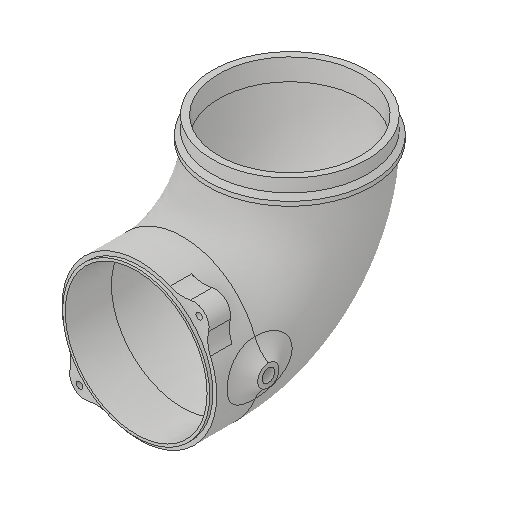
# Autodesk Inventor part: 3DP_PLA_Turbine_exhaust
Saved by Autodesk Inventor 2025 (Build 290162010, 162A)
## iProperties
Created: 2020-03-29
Part Number: 3DP_PLA_Turbine_exhaust
Material: Generic
Document SubType Name: Modeling
Designer: Andrzej
Density: 1 g/cm^3
Appearance: Default
Author: Andrzej
Autodesk Inventor part; units mm, degrees
ref_plane "XZ Plane" through (0, 0, 0) normal (0, 1, 0) x (-1, 0, 0)
ref_plane "XY Plane" through (0, 0, 0) normal (0, 0, 1) x (1, 0, 0)
sketch "Sketch1" plane through (0, 0, 0) normal (0, 0, 1) x (1, 0, 0)
  circle A0 centre (0, 0) radius 33
  circle A1 centre (0, 0) radius 36
  circle A2 centre (0, 0) radius 34.2
  dimension "d0" = 66
  dimension "d1" = 3
  dimension "d2" = 68.4
  constraints: 3 centre point, 2 coincident
  measures "d0" diameter of A0
  measures "d1" radial gap between concentric circles of A0 A1
  measures "d2" diameter of A2
extrude "Extrusion1" add sketch "Sketch1" along normal blind 1.5 contours A2
sketch "Sketch4" plane through (0, 0, 0) normal (1, 0, 0) x (0, 1, 0)
  line L0 (0, 0) -> (0, -20)
  line L1 (50, -70) -> (60, -70)
  arc A0 (0, -20) -> (50, -70) centre (50, -20) ccw
  dimension "d10" = 20
  dimension "d11" = 10
  dimension "d12" = 50
  dimension "d13" = 50
  dimension "d14" = 50
  constraints: 4 end point, 2 point on circle, 1 centre point, 1 horizontal, 1 vertical
  measures "d10" distance of L0.start L0.end
  measures "d11" distance of L1.start L1.end
  measures "d12" horizontal distance of L1.start L0.end
  measures "d13" horizontal distance of L1.start L0.end
  measures "d14" radius of A0
sweep "Sweep1" add profiles "Sketch1" path "Sketch4" path curves L0 A0 L1 contours A1 | A2
sketch "Sketch5" plane through (0, 0, 0) normal (0, 0, 1) x (1, 0, 0)
  circle A0 centre (0, 0) radius 36 projected
  circle A1 centre (0, 0) radius 34.2 projected
  line L0 (0, 0) -> (27.8105, 27.8105)
  line L1 (0, 0) -> (89.128, 0) construction
  line L2 (0, 0) -> (-27.8105, -27.8105)
  line L3 (0, 0) -> (71.454, 0) construction
  circle A2 centre (0, 0) radius 39.33
  circle A3 centre (27.8105, 27.8105) radius 1.5
  circle A4 centre (-27.8105, -27.8105) radius 1.5
  circle A5 centre (0, 0) radius 36 projected
  arc A6 (-29.9009, -20.0483) -> (-20.0483, -29.9009) centre (-25.4558, -25.4558) ccw
  arc A7 (29.9009, 20.0483) -> (20.0483, 29.9009) centre (25.4558, 25.4558) ccw
  dimension "d18" = 45
  dimension "d20" = 135
  dimension "d21" = 78.66
  dimension "d22" = 3
  dimension "d23" = 3
  dimension "d26" = 7
  dimension "d27" = 7
  constraints: 12 point on circle, 8 end point, 5 centre point, 3 coincident, 2 horizontal, 2 point on line
  measures "d18" angle of L1 L0
  measures "d20" angle of L2 L3
  measures "d21" diameter of A2
  measures "d22" diameter of A3
  measures "d23" diameter of A4
  measures "d26" radius of A6
  measures "d27" radius of A7
extrude "Extrusion3" add sketch "Sketch5" against normal blind 10 contours A0 L0 A3 A2 A7 | A6 A2 A4 L2 A0 | A0 A7 A2 A3 L0 | A2 A3 A7 | L2 A4 A2 A6 A0 | A6 A2 A4
fillet "Fillet1" radius 15 4 edges at (29.9009, 20.0483, -5) (20.0483, 29.9009, -5) (-29.9009, -20.0483, -5) (-20.0483, -29.9009, -5)
ref_plane "Work Plane1" through (40, 0, 0) normal (1, 0, 0) x (0, 1, 0)
sketch "Sketch6" plane through (40, 0, 0) normal (1, 0, 0) x (0, 1, 0)
  line L0 (-33, -20) -> (33, -20) projected
  circle A0 centre (0, -20) radius 3
  circle A1 centre (0, -20) radius 5
  point P0 (0, 0)
  dimension "d32" = 6
  dimension "d33" = 2
  constraints: 2 centre point, 1 midpoint
  measures "d32" diameter of A0
  measures "d33" radial gap between concentric circles of A0 A1
extrude "Extrusion4" cut sketch "Sketch6" against normal blind 10 contours A0 L0 | L0 A0
extrude "Extrusion5" add sketch "Sketch6" against normal blind 5 contours A0 L0 A1 | L0 A1 A0
fillet "Fillet2" radius 15 4 edges at (35.8299, 3.6235, -23.4453) (35.8227, -3.4461, -23.6227) (35.7977, -3.8113, -16.7636) (35.7975, 3.8128, -16.7655)
ref_plane "Work Plane2" through (0, 52, -70) normal (0, 1, 0) x (1, 0, 0)
sketch "Sketch7" plane through (0, 52, -70) normal (0, 1, 0) x (1, 0, 0)
  circle A0 centre (0, 0) radius 36 projected
  circle A1 centre (0, 0) radius 38
  point P0 (0, -70)
  dimension "d40" = 2
  constraints: 1 centre point
  measures "d40" radial gap between concentric circles of A0 A1
extrude "Extrusion6" add sketch "Sketch7" against normal blind 2
chamfer "Chamfer1" distance 2 angle 45 1 edges at (-36, 52, -70)
equation "\"d13\" = d12"
equation "\"d14\" = d12"
body "Solid1"
